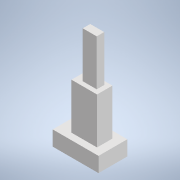
# Autodesk Inventor part: 2nd model
Saved by Autodesk Inventor 2020 (Build 240168000, 168)
## iProperties
Created: 2020-01-19
Part Number: 2nd model
Material: Generic
Document SubType Name: Modeling
Designer: admin
Density: 1 g/cm^3
Appearance: Default
Author: admin
Autodesk Inventor part; units mm, degrees
ref_plane "YZ Plane" through (0, 0, 0) normal (1, 0, 0) x (0, 1, 0)
ref_plane "XZ Plane" through (0, 0, 0) normal (0, 1, 0) x (-1, 0, 0)
ref_plane "XY Plane" through (0, 0, 0) normal (0, 0, 1) x (1, 0, 0)
sketch "Sketch1" plane through (0, 0, 0) normal (1, 0, 0) x (0, 1, 0)
  line L0 (10.236, 20.6024) -> (1.9777, 20.6024)
  line L1 (1.9777, 20.6024) -> (1.9777, 4.6508)
  line L2 (1.9777, 4.6508) -> (10.236, 4.6508)
  line L3 (10.236, 4.6508) -> (10.236, 20.6024)
  point P0 (0, 0)
  constraints: 8 end point, 2 parallel, 1 horizontal, 1 perpendicular
extrude "Extrusion1" add sketch "Sketch1" along normal blind 25.4
sketch "Sketch2" plane through (0, 10.236, 20.6024) normal (0, 1, 0) x (1, 0, 0)
  line L0 (6.7613, 3.64) -> (20.9369, 3.64)
  line L1 (20.9369, 3.64) -> (20.9369, 12.1675)
  line L2 (20.9369, 12.1675) -> (6.7613, 12.1675)
  line L3 (6.7613, 12.1675) -> (6.7613, 3.64)
  line L4 (10.89, 6.1434) -> (17.4809, 6.1434)
  line L5 (17.4809, 6.1434) -> (17.4809, 9.7454)
  line L6 (17.4809, 9.7454) -> (11.2732, 9.7454)
  line L7 (11.2732, 9.7454) -> (11.2732, 6.1434)
  point P0 (0, 20.6024)
  constraints: 16 end point, 4 perpendicular, 2 horizontal, 2 parallel, 1 point on line
extrude "Extrusion2" add sketch "Sketch2" along normal blind 25.4 contours L3 L2 L1 L0 | L7 L6 L5 L4
sketch "Sketch3" plane through (0, 35.636, 20.6024) normal (0, 1, 0) x (1, 0, 0)
  line L0 (10.6145, 6.041) -> (18.3551, 6.041)
  line L1 (18.3551, 6.041) -> (18.3551, 10.1795)
  line L2 (18.3551, 10.1795) -> (10.6145, 10.1795)
  line L3 (10.6145, 10.1795) -> (10.6145, 6.041)
  point P0 (0, 20.6024)
  constraints: 8 end point, 2 parallel, 1 horizontal, 1 perpendicular
extrude "Extrusion3" add sketch "Sketch3" along normal blind 25.4
body "Solid1"
